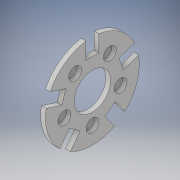
# Autodesk Inventor part: Magnetic Disk
Saved by Autodesk Inventor 2019 (Build 230136000, 136)
## iProperties
Created: 2020-12-02
Part Number: Magnetic Disk
Material: Generic
Document SubType Name: Modeling
Designer: infinity
Density: 1 g/cm^3
Appearance: Default
Author: infinity
Autodesk Inventor part; units mm, degrees
ref_plane "YZ Plane" through (0, 0, 0) normal (1, 0, 0) x (0, 1, 0)
ref_plane "XZ Plane" through (0, 0, 0) normal (0, 1, 0) x (-1, 0, 0)
ref_plane "XY Plane" through (0, 0, 0) normal (0, 0, 1) x (1, 0, 0)
sketch "Sketch1" plane through (0, 0, 0) normal (1, 0, 0) x (0, 1, 0)
  circle A0 centre (0, 0) radius 22.25
  circle A1 centre (0, 0) radius 8.625
  line L0 (8.625, 0) -> (22.25, 0) construction
  line L1 (21.91, 3.875) -> (7.7055, 3.875) construction
  line L2 (7.7055, -3.875) -> (21.91, -3.875) construction
  circle A2 centre (-14, 0) radius 3.0375
  circle A3 centre (-4.3262, -13.3148) radius 3.0375
  circle A4 centre (11.3262, -8.229) radius 3.0375
  circle A5 centre (11.3262, 8.229) radius 3.0375
  circle A6 centre (-4.3262, 13.3148) radius 3.0375
  dimension "d0" = 44.5
  dimension "d1" = 17.25
  dimension "d2" = 7.75
  dimension "d3" = 3.875
  dimension "d4" = 0
  dimension "d5" = 6.075
  dimension "d32" = 14
  dimension "d35" = 360
  constraints: 7 centre point, 6 end point, 6 point on circle, 2 coincident, 2 horizontal, 1 parallel, 1 point on line, 11 other
  measures "d0" diameter of A0
  measures "d1" diameter of A1
  measures "d2" distance between parallel lines of L2 L1
  measures "d3" distance between parallel lines of L0 L1
  measures "d4" distance from line of point (0, 0) L0
  measures "d5" diameter of A2
  measures "d32" distance of A2.centre point (0, 0)
extrude "Extrusion1" add sketch "Sketch1" along normal blind 2
sketch "Sketch2" plane through (0, 0, 0) normal (-1, 0, 0) x (0, 0, 1)
  circle A0 centre (0, 0) radius 8.625 projected
  circle A1 centre (0, 0) radius 22.25 projected
  constraints: 2 centre point
extrude "Extrusion2" add sketch "Sketch2" along normal blind 0.25
sketch "Sketch3" plane through (2, 0, 0) normal (1, 0, 0) x (0, 0, -1)
  line L0 (-3.1, 26.8099) -> (3.1, 26.8099)
  line L1 (3.1, 26.8099) -> (3.1, 14.25)
  line L2 (3.1, 14.25) -> (-3.1, 14.25)
  line L3 (-3.1, 14.25) -> (-3.1, 26.8099)
  circle A0 centre (0, 0) radius 22.25 construction
  line L4 (-2.05, 26.8099) -> (2.05, 26.8099)
  line L5 (2.05, 26.8099) -> (2.05, 14.25)
  line L6 (2.05, 14.25) -> (-2.05, 14.25)
  line L7 (-2.05, 14.25) -> (-2.05, 26.8099)
  line L8 (-26.4557, 5.3365) -> (-24.5398, 11.233)
  line L9 (-24.5398, 11.233) -> (-12.5946, 7.3518)
  line L10 (-12.5946, 7.3518) -> (-14.5105, 1.4552)
  line L11 (-14.5105, 1.4552) -> (-26.4557, 5.3365)
  line L12 (-26.1313, 6.3351) -> (-24.8643, 10.2344)
  line L13 (-24.8643, 10.2344) -> (-12.9191, 6.3532)
  line L14 (-12.9191, 6.3532) -> (-14.186, 2.4538)
  line L15 (-14.186, 2.4538) -> (-26.1313, 6.3351)
  line L16 (-13.2505, -23.5118) -> (-18.2664, -19.8676)
  line L17 (-18.2664, -19.8676) -> (-10.8839, -9.7064)
  line L18 (-10.8839, -9.7064) -> (-5.868, -13.3506)
  line L19 (-5.868, -13.3506) -> (-13.2505, -23.5118)
  line L20 (-14.1, -22.8947) -> (-17.417, -20.4847)
  line L21 (-17.417, -20.4847) -> (-10.0344, -10.3235)
  line L22 (-10.0344, -10.3235) -> (-6.7175, -12.7335)
  line L23 (-6.7175, -12.7335) -> (-14.1, -22.8947)
  line L24 (18.2664, -19.8676) -> (13.2505, -23.5118)
  line L25 (13.2505, -23.5118) -> (5.868, -13.3506)
  line L26 (5.868, -13.3506) -> (10.8839, -9.7064)
  line L27 (10.8839, -9.7064) -> (18.2664, -19.8676)
  line L28 (17.417, -20.4847) -> (14.1, -22.8947)
  line L29 (14.1, -22.8947) -> (6.7175, -12.7335)
  line L30 (6.7175, -12.7335) -> (10.0344, -10.3235)
  line L31 (10.0344, -10.3235) -> (17.417, -20.4847)
  line L32 (24.5398, 11.233) -> (26.4557, 5.3365)
  line L33 (26.4557, 5.3365) -> (14.5105, 1.4552)
  line L34 (14.5105, 1.4552) -> (12.5946, 7.3518)
  line L35 (12.5946, 7.3518) -> (24.5398, 11.233)
  line L36 (24.8643, 10.2344) -> (26.1313, 6.3351)
  line L37 (26.1313, 6.3351) -> (14.186, 2.4538)
  line L38 (14.186, 2.4538) -> (12.9191, 6.3532)
  line L39 (12.9191, 6.3532) -> (24.8643, 10.2344)
  dimension "d15" = 6.2
  dimension "d16" = 3.1
  dimension "d17" = 8
  dimension "d22" = 0
  dimension "d23" = 0
  dimension "d24" = 1.05
  dimension "d25" = 1.05
  dimension "d28" = 360
  constraints: 80 end point, 4 parallel, 2 horizontal, 2 perpendicular, 81 other
  measures "d15" distance of L0.start L0.end
  measures "d16" distance from line of point (0, 0) L3
  measures "d17" distance edge to line of A0 L2
  measures "d22" distance between parallel lines of L0 L4
  measures "d23" distance between parallel lines of L2 L6
  measures "d24" distance between parallel lines of L3 L7
  measures "d25" distance between parallel lines of L1 L5
extrude "Extrusion3" cut sketch "Sketch3" against normal up to surface (2.25 mm away)
equation "\"d3\" = 0.5 * d2"
equation "\"d16\" = 0.5 * d15"
equation "\"d25\" = d24"
body "Solid1"
